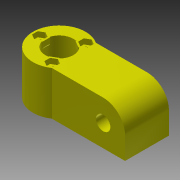
# Autodesk Inventor part: SHOULDER
Saved by Autodesk Inventor 2013 (Build 170138000, 138)
## iProperties
Created: 2013-11-19
Part Number: SHOULDER
Material: Generic
Document SubType Name: Modeling
Designer: employee
Density: 1 g/cm^3
Author: employee
Autodesk Inventor part; units mm, degrees
ref_plane "YZ Plane" through (0, 0, 0) normal (1, 0, 0) x (0, 1, 0)
ref_plane "XZ Plane" through (0, 0, 0) normal (0, 1, 0) x (-1, 0, 0)
ref_plane "XY Plane" through (0, 0, 0) normal (0, 0, 1) x (1, 0, 0)
sketch "Sketch1" plane through (0, 0, 0) normal (0, 0, 1) x (1, 0, 0)
  circle A0 centre (0, 0) radius 9.625
  arc A1 (0, 12.5) -> (0, -12.5) centre (0, 0) ccw
  line L0 (0, -12.5) -> (37.5, -12.5)
  line L1 (37.5, -12.5) -> (37.5, 12.5)
  line L2 (37.5, 12.5) -> (0, 12.5)
  line L3 (37.5, 0) -> (9.625, 0) construction
  dimension "d0" = 19.25
  dimension "d2" = 25
  dimension "d4" = 37.5
  constraints: 8 end point, 2 coincident, 2 horizontal, 2 point on circle, 2 tangent, 1 centre point, 1 horizontal alignment, 1 midpoint, 1 parallel, 1 perpendicular, 2 other
  measures "d2" diameter of A1
  measures "d4" distance of L3.start point (0, 0)
extrude "Extrusion1" add sketch "Sketch1" along normal blind 25
sketch "Sketch2" plane through (0, -12.5, 0) normal (0, -1, 0) x (1, 0, 0)
  line L0 (37.5, 0) -> (37.5, 25) projected
  line L1 (0, 25) -> (37.5, 25) projected
  line L2 (0, 0) -> (0, 25) projected
  line L3 (37.5, 0) -> (50, 0)
  line L4 (50, 0) -> (50, 12.5)
  arc A0 (50, 12.5) -> (37.5, 25) centre (37.5, 12.5) ccw
  constraints: 4 end point, 2 perpendicular, 2 point on circle, 2 tangent, 1 centre point, 1 coincident, 1 midpoint
extrude "Extrusion2" add sketch "Sketch2" against normal up to surface (25 mm away)
sketch "Sketch3" plane through (0, -12.5, 0) normal (0, -1, 0) x (1, 0, 0)
  arc A0 (50, 12.5) -> (37.5, 25) centre (37.5, 12.5) ccw projected
  circle A1 centre (37.5, 12.5) radius 4.1
  dimension "d9" = 8.2
  constraints: 1 centre point, 1 coincident
  measures "d9" diameter of A1
extrude "Extrusion3" cut sketch "Sketch3" against normal through all
sketch "Sketch10" plane through (50, 12.5, 12.5) normal (0, 1, 0) x (1, 0, 0)
  circle A0 centre (-12.5, 0) radius 4.1 projected
  line L0 (-20.121, 0) -> (-16.3105, 6.6)
  line L1 (-16.3105, 6.6) -> (-8.6895, 6.6)
  line L2 (-8.6895, 6.6) -> (-4.879, 0)
  line L3 (-4.879, 0) -> (-8.6895, -6.6)
  line L4 (-8.6895, -6.6) -> (-16.3105, -6.6)
  line L5 (-16.3105, -6.6) -> (-20.121, 0)
  point P0 (-50, 12.5)
  point P1 (-12.5, 6.6)
  dimension "d47" = 13.2
  constraints: 12 end point, 1 coincident, 1 horizontal alignment, 1 midpoint, 13 other
  measures "d47" distance between parallel lines of L4 L1
extrude "Extrusion10" cut sketch "Sketch10" against normal blind 8
sketch "Sketch11" plane through (0, 0, 0) normal (0, 0, -1) x (-1, 0, 0)
  circle A0 centre (0, 0) radius 9.625 projected
  arc A1 (0, -12.5) -> (0, 12.5) centre (0, 0) ccw projected
  circle A2 centre (0, 0) radius 19.05
  dimension "d50" = 38.1
  constraints: 1 centre point, 1 coincident
  measures "d50" diameter of A2
extrude "Extrusion11" add sketch "Sketch11" against normal up to surface (25 mm away)
sketch "Sketch12" plane through (0, 0, 0) normal (0, 0, -1) x (-1, 0, 0)
  arc A0 (-14.3754, -12.5) -> (-14.3754, 12.5) centre (0, 0) ccw projected
  circle A1 centre (14.2875, 0) radius 1.6
  dimension "d55" = 14.2875
  dimension "d56" = 3.2
  constraints: 1 centre point, 1 horizontal alignment
  measures "d55" distance of A1.centre A0.centre
  measures "d56" diameter of A1
extrude "Extrusion12" cut sketch "Sketch12" against normal through all
sketch "Sketch13" plane through (0, 0, 25) normal (0, 0, 1) x (1, 0, 0)
  circle A0 centre (-14.2875, 0) radius 1.6 projected
  line L0 (-14.2875, 3.262) -> (-11.4625, 1.631)
  line L1 (-11.4625, 1.631) -> (-11.4625, -1.631)
  line L2 (-11.4625, -1.631) -> (-14.2875, -3.262)
  line L3 (-14.2875, -3.262) -> (-17.1125, -1.631)
  line L4 (-17.1125, -1.631) -> (-17.1125, 1.631)
  line L5 (-17.1125, 1.631) -> (-14.2875, 3.262)
  dimension "d59" = 5.65
  constraints: 12 end point, 1 coincident, 1 vertical, 13 other
  measures "d59" distance between parallel lines of L1 L4
extrude "Extrusion13" cut sketch "Sketch13" against normal blind 3
pattern_circular "Circular Pattern3" count 3 over 360 about axis through (0, 0, 0) along (0, 0, 1) of "Extrusion13", "Extrusion12"
body "Solid1"
